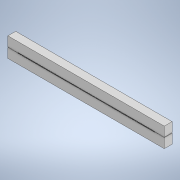
# Autodesk Inventor part: SLASlotDieWireInsertedSiCMonofilamentHolder
Saved by Autodesk Inventor 2021 (Build 250183000, 183)
## iProperties
Created: 2021-11-04
Part Number: SLASlotDieWireInsertedSiCMonofilamentHolder
Material: Generic
Document SubType Name: Sheet Metal
Designer: Unit-005
Density: 1 g/cm^3
Sheet Metal Rule: Default
Appearance: Default
Author: Unit-005
Autodesk Inventor part; units mm, degrees
ref_plane "YZ Plane" through (0, 0, 0) normal (1, 0, 0) x (0, 1, 0)
ref_plane "XZ Plane" through (0, 0, 0) normal (0, 1, 0) x (-1, 0, 0)
ref_plane "XY Plane" through (0, 0, 0) normal (0, 0, 1) x (1, 0, 0)
sketch "Sketch1" plane through (0, 0, 0) normal (0, 0, 1) x (1, 0, 0)
  line L0 (-50, 6.25) -> (50, 6.25)
  line L1 (50, 6.25) -> (50, -6.25)
  line L2 (50, -6.25) -> (-50, -6.25)
  line L3 (-50, -6.25) -> (-50, 6.25)
  line L4 (-50, 6.25) -> (50, -6.25) construction
  line L5 (50, 6.25) -> (-50, -6.25) construction
  line L6 (-50, 0.15) -> (50, 0.15)
  line L7 (50, 0.15) -> (50, -0.15)
  line L8 (50, -0.15) -> (-50, -0.15)
  line L9 (-50, -0.15) -> (-50, 0.15)
  line L10 (-50, 0.15) -> (50, -0.15) construction
  line L11 (50, 0.15) -> (-50, -0.15) construction
  point P0 (0, 0)
  dimension "d0" = 100
  dimension "d1" = 12.5
  dimension "d2" = 0.3
  constraints: 24 end point, 4 midpoint, 4 parallel, 2 horizontal, 2 perpendicular, 1 point on line
  measures "d0" distance of L1.end L2.end
  measures "d1" distance of L0.end L1.end
  measures "d2" distance of L6.end L7.end
extrude "Extrusion1" add sketch "Sketch1" along normal blind 5 contours L0 L1 L6 L3 | L8 L1 L2 L3
sketch "Sketch3" plane through (0, 0, 0) normal (0, 0, 1) x (1, 0, 0)
  line L0 (50, -6.25) -> (50, -0.15) projected
  line L1 (-50, -6.25) -> (50, -6.25) projected
  line L2 (-50, -0.15) -> (-50, -6.25) projected
  line L3 (50, -0.15) -> (-50, -0.15) projected
  line L4 (-50, 6.25) -> (-50, 0.15) projected
  line L5 (50, 6.25) -> (-50, 6.25) projected
  line L6 (50, 0.15) -> (50, 6.25) projected
  line L7 (-50, 0.15) -> (50, 0.15) projected
  line L8 (-70, 0) -> (70, 0) projected
  line L9 (0, -8.75) -> (0, 8.75) projected
  line L10 (-0.125, -0.275) -> (0.125, -0.275)
  line L11 (0.125, -0.275) -> (0.125, 0.275)
  line L12 (0.125, 0.275) -> (-0.125, 0.275)
  line L13 (-0.125, 0.275) -> (-0.125, -0.275)
  line L14 (-0.125, -0.275) -> (0.125, 0.275) construction
  line L15 (0.125, -0.275) -> (-0.125, 0.275) construction
  point P0 (0, 0)
  dimension "d9" = 0.25
  dimension "d11" = 0.125
  constraints: 12 end point, 2 midpoint, 2 parallel, 1 horizontal, 1 perpendicular
  measures "d9" distance of L12.end L11.end
  measures "d11" distance between parallel lines of L3 L10
extrude "Extrusion3" cut sketch "Sketch3" along normal through all contours L11 L10 L9 L3 | L3 L9 L8 L11 | L10 L13 L3 L9 | L3 L13 L8 L9 | L8 L9 L7 L11 | L8 L13 L7 L9 | L7 L9 L12 L11 | L7 L13 L12 L9
pattern_linear "Rectangular Pattern1" count 175 spacing 0.5 along (1, 0, 0) of "Extrusion3" first direction both ways yes
equation "\"BendRadius\" = Thickness"
equation "\"BendReliefWidth\" = Thickness"
equation "\"BendReliefDepth\" = 0.5 * Thickness"
equation "\"CornerReliefSize\" = 4 * Thickness"
equation "\"MinimumRemnant\" = 2 * Thickness"
equation "\"TransitionRadius\" = BendRadius"
equation "\"JacobiRadiusSize\" = BendRadius"
equation "\"GapSize\" = Thickness"
equation "\"Thickness\" = 3.048"
body "Solid1"
